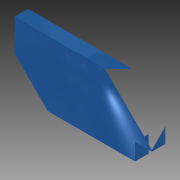
# Autodesk Inventor part: ZAxisNutMount
Saved by Autodesk Inventor 2015 SP1 (Build 190203100, 203)
## iProperties
Created: 2014-12-11
Part Number: ZAxisNutMount
Material: Generic
Document SubType Name: Modeling
Designer: Jack
Density: 1 g/cm^3
Appearance: Cyan
Author: Jack
Autodesk Inventor part; units mm, degrees
ref_plane "YZ Plane" through (0, 0, 0) normal (1, 0, 0) x (0, 1, 0)
ref_plane "XZ Plane" through (0, 0, 0) normal (0, 1, 0) x (-1, 0, 0)
ref_plane "XY Plane" through (0, 0, 0) normal (0, 0, 1) x (1, 0, 0)
sketch "Sketch1" plane through (0, 0, 0) normal (0, 0, 1) x (1, 0, 0)
  line L0 (0, 0) -> (122, 0)
  line L1 (122, 0) -> (122, 12)
  line L2 (122, 12) -> (0, 12)
  line L3 (0, 12) -> (0, 0)
  dimension "d0" = 122
  dimension "d1" = 12
  constraints: 8 end point, 2 parallel, 1 horizontal, 1 perpendicular
  measures "d0" distance of L2.end L1.end
  measures "d1" distance of L2.end L0.start
extrude "Extrusion1" add sketch "Sketch1" along normal blind 58
sketch "Sketch2" plane through (0, 12, 0) normal (0, 1, 0) x (1, 0, 0)
  line L0 (122, 0) -> (0, 0) projected
  line L1 (0, 0) -> (0, -58) projected
  line L2 (0, -28) -> (15, -28)
  line L3 (15, -28) -> (15, 0)
  line L4 (0, 0) -> (122, 0) projected
  line L5 (122, 0) -> (122, -58) projected
  line L6 (122, -28) -> (107, -28)
  line L7 (107, -28) -> (107, 0)
  dimension "d4" = 28
  dimension "d5" = 15
  constraints: 8 end point, 6 point on line, 2 perpendicular, 1 collinear, 1 horizontal
  measures "d4" distance of L6.end L7.end
  measures "d5" distance of L6.start L6.end
extrude "Extrusion2" cut sketch "Sketch2" against normal up to next
body "Solid1"
